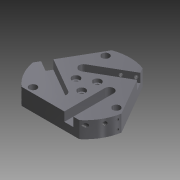
# Autodesk Inventor part: Tool Turret Disk
Saved by Autodesk Inventor 2011 SP1 (Build 150282100, 282)
## iProperties
Created: 2011-10-17
Part Number: Tool Turret Disk
Document SubType Name: Modeling
Designer: James
Density: 1 g/cm^3
Author: James
Autodesk Inventor part; units mm, degrees
note: some values were not read from the file. Chosen so that the rebuilt part matches the saved one: direction of "Hole4"; direction of "Hole5".
ref_plane "YZ Plane" through (0, 0, 0) normal (1, 0, 0) x (0, 1, 0)
sketch "Sketch1" plane through (0, 0, 0) normal (0, 0, 1) x (1, 0, 0)
  line L0 (-20.6036, 56.3515) -> (-59.1036, -10.3325)
  line L1 (20.6036, 56.3515) -> (59.1038, -10.3328)
  line L2 (-38.5, -46.019) -> (38.5004, -46.019)
  arc A0 (20.6036, 56.3515) -> (-20.6036, 56.3515) centre (0, 0) ccw
  arc A1 (-59.1036, -10.3325) -> (-38.5, -46.019) centre (0, 0) ccw
  arc A2 (38.5004, -46.019) -> (59.1038, -10.3328) centre (0, 0) ccw
  line L3 (0, 0) -> (0, 24.8035)
  dimension "d3" = 60
  dimension "d5" = 60
  dimension "d6" = 90
  dimension "d55" = 46.019
  dimension "d56" = 46.019
  dimension "d57" = 46.019
  dimension "d58" = 60
  dimension "d59" = 60
  dimension "d60" = 60.0003
  constraints: 8 end point, 6 point on circle, 3 centre point, 1 coincident, 1 vertical
  measures "d3" angle of L1 L0
  measures "d5" angle of L2 L0
  measures "d6" angle of L2 L3
  measures "d55" distance from line of L0 point (0, 0)
  measures "d56" distance from line of L1 point (0, 0)
  measures "d57" distance from line of L2 point (0, 0)
  measures "d58" radius of A0
  measures "d59" radius of A1
  measures "d60" radius of A2
extrude "Extrusion1" add sketch "Sketch1" along normal blind 22
sketch "Sketch3" plane through (0, 0, 0) normal (0, 0, -1) x (-1, 0, 0)
  circle A0 centre (0, 0) radius 7.5 projected
  arc A1 (38.5, -46.019) -> (59.1036, -10.3325) centre (0, 0) ccw projected
  circle A2 centre (0, 0) radius 20
  dimension "d12" = 40
  constraints: 1 centre point, 1 coincident
  measures "d12" diameter of A2
extrude "Extrusion3" add sketch "Sketch3" along normal blind 0.3
sketch "Sketch4" plane through (0, 0, 0) normal (0, 0, -1) x (-1, 0, 0)
  circle A0 centre (0, 0) radius 7.5 projected
  circle A1 centre (0, 0) radius 7.5
  constraints: 1 centre point, 1 coincident, 1 concentric
extrude "Extrusion4" cut sketch "Sketch4" against normal blind 10
sketch "Sketch5" plane through (0, 0, 22) normal (0, 0, 1) x (1, 0, 0)
  arc A0 (20.6036, 56.3515) -> (-20.6036, 56.3515) centre (0, 0) ccw projected
  arc A1 (-59.1036, -10.3325) -> (-38.5, -46.019) centre (0, 0) ccw projected
  line L0 (38.5004, -46.019) -> (-38.5, -46.019) projected
  line L1 (0, 0) -> (0.0002, -46.019) construction
  line L2 (0, 0) -> (-31.1428, -0.0001) construction
  point P0 (-12.041, -0.0001)
  dimension "d91" = 12.041
  constraints: 4 end point, 1 midpoint, 1 perpendicular, 1 point on line
  measures "d91" distance of A0.centre point (-12.041, 0)
hole "Hole1" at (-12.041, -0.0001, 22) direction (0, 0, -1) diameter 6.5 end through all counterbore diameter 10.4 counterbore depth 4.8 clearance for "Hex Head Cap Screw ISO 24017" size "M6" standard "ISO"
pattern_circular "Circular Pattern1" count 3 over 360 about axis through (0, 0, 0) along (0, 0, 1) of "Hole1"
sketch "Sketch6" plane through (0, 0, 22) normal (0, 0, 1) x (1, 0, 0)
  line L0 (38.5004, -46.019) -> (-38.5, -46.019) projected
  line L1 (30.5, -46.019) -> (30.5, 7.981)
  line L2 (18.5, 7.981) -> (18.5, -46.019)
  arc A0 (30.5, 7.981) -> (18.5, 7.981) centre (24.5, 7.981) ccw
  line L3 (18.5, -46.019) -> (30.5, -46.019)
  dimension "d61" = 57
  dimension "d62" = 12
  constraints: 6 end point, 2 perpendicular, 2 point on circle, 2 point on line, 1 centre point, 1 collinear
  measures "d61" distance from line of L2 L0.end
  measures "d62" distance between parallel lines of L1 L2
extrude "Extrusion5" cut sketch "Sketch6" against normal blind 12
pattern_circular "Circular Pattern2" count 3 over 360 about axis through (0, 0, 0) along (0, 0, 1) of "Extrusion5"
sketch "Sketch7" plane through (0, 0, 22) normal (0, 0, 1) x (1, 0, 0)
  arc A0 (-59.1036, -10.3325) -> (-38.5, -46.019) centre (0, 0) ccw projected
  line L0 (38.5004, -46.019) -> (30.5, -46.019) projected
  line L1 (18.5, -46.019) -> (30.5, -46.019) construction
  line L2 (24.6036, 49.4233) -> (30.6036, 39.031) construction
  line L3 (-55.1036, -3.4043) -> (-49.1036, 6.988) construction
  arc A1 (38.5004, -46.019) -> (59.1038, -10.3328) centre (0, 0) ccw projected
  line L4 (0, 0) -> (30.6036, 39.031) construction
  line L5 (0, 0) -> (18.5, -46.019) construction
  line L6 (0, 0) -> (-49.1036, 6.988) construction
  line L7 (0, 0) -> (-36.8251, 91.6031) construction
  line L8 (0, 0) -> (-45.2166, -57.6679) construction
  line L9 (0, 0) -> (86.2103, -12.2688) construction
  point P0 (-18.4126, 45.8016)
  dimension "d63" = 60
  dimension "d64" = 60
  dimension "d65" = 60
  dimension "d66" = 49.364
  constraints: 18 end point, 1 collinear, 1 midpoint
  measures "d63" angle of L7 L4
  measures "d64" angle of L4 L9
  measures "d65" angle of L8 L5
  measures "d66" distance of A0.centre point (-18.413, 45.802)
hole "Hole2" at (-18.4126, 45.8016, 22) direction (0, 0, -1) diameter 10 end through all
pattern_circular "Circular Pattern3" count 3 over 360 about axis through (0, 0, 0) along (0, 0, 1) of "Hole2"
sketch "Sketch9" plane through (0, 0, 22) normal (0, 0, 1) x (1, 0, 0)
  circle A0 centre (48.8716, -6.955) radius 5 projected
  circle A1 centre (-30.459, -38.8465) radius 5 projected
  circle A2 centre (-18.4126, 45.8016) radius 5 projected
  line L0 (-8.3382, -30.4043) -> (-55.1036, -3.4043) projected
  line L1 (-59.1036, -10.3325) -> (-55.1036, -3.4043) projected
  arc A3 (-59.1036, -10.3325) -> (-38.5, -46.019) centre (0, 0) ccw projected
  line L2 (18.5, -46.019) -> (-38.5, -46.019) projected
  line L3 (18.5, -46.019) -> (18.5, 7.981) projected
  arc A4 (30.5, 7.981) -> (18.5, 7.981) centre (24.5, 7.981) ccw projected
  line L4 (30.5, 7.981) -> (30.5, -46.019) projected
  line L5 (38.5004, -46.019) -> (30.5, -46.019) projected
  arc A5 (38.5004, -46.019) -> (59.1038, -10.3328) centre (0, 0) ccw projected
  line L6 (30.6036, 39.031) -> (59.1038, -10.3328) projected
  line L7 (30.6036, 39.031) -> (-16.1617, 12.031) projected
  arc A6 (-22.1617, 22.4233) -> (-16.1617, 12.031) centre (-19.1617, 17.2271) ccw projected
  line L8 (-22.1617, 22.4233) -> (24.6036, 49.4233) projected
  line L9 (20.6036, 56.3515) -> (24.6036, 49.4233) projected
  arc A7 (20.6036, 56.3515) -> (-20.6036, 56.3515) centre (0, 0) ccw projected
  line L10 (-49.1036, 6.988) -> (-20.6036, 56.3515) projected
  line L11 (-49.1036, 6.988) -> (-2.3382, -20.012) projected
  arc A8 (-8.3382, -30.4043) -> (-2.3382, -20.012) centre (-5.3382, -25.2081) ccw projected
  circle A9 centre (10.3923, -6) radius 5.2 projected
  circle A10 centre (-10.3923, -6) radius 5.2 projected
  circle A11 centre (0, 12) radius 5.2 projected
  line L12 (-18.4126, 45.8016) -> (-15.1593, 64.142)
  dimension "d77" = 4
  constraints: 2 end point
  measures "d77" distance from line of L12 L10.end
ref_plane "Work Plane2" through (-15.1593, 64.142, 22) normal (0.1746576, 0.9846292, 0) x (-0.9846292, 0.1746576, 0)
sketch "Sketch11" plane through (-15.1593, 64.142, 22) normal (0.1746576, 0.9846292, 0) x (-0.9846292, 0.1746576, 0)
  line L0 (5, -22) -> (-5, -22) projected
  line L1 (-5, 0) -> (5, 0) projected
  line L2 (0, -22) -> (0, 0) construction
  point P0 (-26.1291, -22)
  point P1 (0, -5.5)
  point P2 (0, -17)
  dimension "d78" = 5.5
  dimension "d79" = 11.5
  constraints: 2 end point, 2 midpoint, 2 point on line
  measures "d78" distance of L2.end point (0, -5.5)
  measures "d79" distance of point (0, -5.5) point (0, -17)
hole "Hole4" at (-15.1593, 64.142, 16.5) at (-15.1593, 64.142, 5) direction (-0.1746576, -0.9846292, 0) diameter 3.242 end up to surface thread size "M4x0.7" class "6H" standard "ISO Metric profile"
pattern_circular "Circular Pattern4" count 3 over 360 about axis through (0, 0, 0) along (0, 0, 1) of "Hole4"
sketch "Sketch12" plane through (0, 0, 22) normal (0, 0, 1) x (1, 0, 0)
  circle A0 centre (48.8716, -6.955) radius 5 projected
  circle A1 centre (-30.459, -38.8465) radius 5 projected
  circle A2 centre (-18.4126, 45.8016) radius 5 projected
  line L0 (-8.3382, -30.4043) -> (-55.1036, -3.4043) projected
  line L1 (-59.1036, -10.3325) -> (-55.1036, -3.4043) projected
  arc A3 (-59.1036, -10.3325) -> (-38.5, -46.019) centre (0, 0) ccw projected
  line L2 (18.5, -46.019) -> (-38.5, -46.019) projected
  line L3 (18.5, -46.019) -> (18.5, 7.981) projected
  arc A4 (30.5, 7.981) -> (18.5, 7.981) centre (24.5, 7.981) ccw projected
  line L4 (30.5, 7.981) -> (30.5, -46.019) projected
  line L5 (38.5004, -46.019) -> (30.5, -46.019) projected
  arc A5 (38.5004, -46.019) -> (59.1038, -10.3328) centre (0, 0) ccw projected
  line L6 (30.6036, 39.031) -> (59.1038, -10.3328) projected
  line L7 (30.6036, 39.031) -> (-16.1617, 12.031) projected
  arc A6 (-22.1617, 22.4233) -> (-16.1617, 12.031) centre (-19.1617, 17.2271) ccw projected
  line L8 (-22.1617, 22.4233) -> (24.6036, 49.4233) projected
  line L9 (20.6036, 56.3515) -> (24.6036, 49.4233) projected
  arc A7 (20.6036, 56.3515) -> (-20.6036, 56.3515) centre (0, 0) ccw projected
  line L10 (-49.1036, 6.988) -> (-20.6036, 56.3515) projected
  line L11 (-49.1036, 6.988) -> (-2.3382, -20.012) projected
  arc A8 (-8.3382, -30.4043) -> (-2.3382, -20.012) centre (-5.3382, -25.2081) ccw projected
  circle A9 centre (6.0205, 10.4278) radius 5.2 projected
  circle A10 centre (6.0205, -10.4278) radius 5.2 projected
  circle A11 centre (-12.041, -0.0001) radius 5.2 projected
  line L12 (30.5, -33.8465) -> (49.5423, -33.8465)
  line L13 (49.5423, -33.8465) -> (59.1038, -33.8465)
  constraints: 4 end point, 1 collinear, 1 parallel, 1 point on circle, 1 point on line
ref_plane "Work Plane3" through (59.1038, -33.8465, 22) normal (1, 0, 0) x (0, 1, 0)
sketch "Sketch13" plane through (59.1038, -33.8465, 22) normal (1, 0, 0) x (0, 1, 0)
  line L0 (-14.6097, -6) -> (10.8842, -6) construction
  line L1 (-12.1725, 0) -> (23.5137, 0) projected
  line L2 (-12.1725, -22) -> (-12.1725, 0) projected
  point P0 (33.8465, -22)
  point P1 (-8.1725, -6)
  point P2 (6.8275, -6)
  dimension "d92" = 6
  dimension "d93" = 4
  dimension "d94" = 15
  constraints: 2 end point, 2 point on line, 1 horizontal
  measures "d92" distance between parallel lines of L0 L1
  measures "d93" distance from line of point (-8.172, -6) L2
  measures "d94" distance of point (6.828, -6) point (-8.172, -6)
hole "Hole5" at (59.1038, -42.019, 16) at (59.1038, -27.019, 16) direction (-1, 0, 0) diameter 4.917 end up to surface thread size "M6x1" class "6H" standard "ISO Metric profile"
pattern_circular "Circular Pattern5" count 3 over 360 about axis through (0, 0, 0) along (0, 0, 1) of "Hole5"
body "Solid1"
